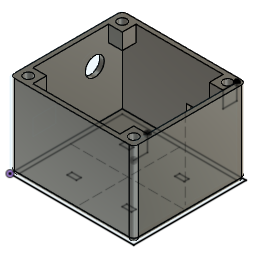
LedstripBox (Autodesk Fusion 360 design; units mm, degrees)
Autodesk Fusion 360 part; units mm, degrees
sketch "Esquisse1" plane through (0, 0, 0) normal (0, 0, 1) x (1, 0, 0)
  line L0 (0, 0) -> (54, 0)
  line L1 (54, 0) -> (54, 49)
  line L2 (54, 49) -> (0, 49)
  line L3 (0, 49) -> (0, 0)
  line L4 (2, 47) -> (52, 47)
  line L5 (52, 47) -> (52, 2)
  line L6 (52, 2) -> (2, 2)
  line L7 (2, 2) -> (2, 47)
  line L8 (13, 37) -> (17, 37)
  line L9 (17, 37) -> (17, 35)
  line L10 (17, 35) -> (13, 35)
  line L11 (13, 35) -> (13, 37)
  line L12 (27, 47) -> (27, 2) construction
  line L13 (2, 24.5) -> (52, 24.5) construction
  line L14 (41, 37) -> (37, 37)
  line L15 (37, 37) -> (37, 35)
  line L16 (37, 35) -> (41, 35)
  line L17 (41, 35) -> (41, 37)
  line L18 (13, 12) -> (17, 12)
  line L19 (13, 14) -> (13, 12)
  line L20 (17, 14) -> (13, 14)
  line L21 (17, 12) -> (17, 14)
  line L22 (37, 12) -> (37, 14)
  line L23 (41, 12) -> (37, 12)
  line L24 (41, 14) -> (41, 12)
  line L25 (37, 14) -> (41, 14)
  dimension "d4" = 54
  dimension "d5" = 49
  dimension "d6" = 2
  dimension "d7" = 2
  dimension "d8" = 2
  dimension "d9" = 2
  dimension "d10" = 4
  dimension "d11" = 2
  dimension "d12" = 10
  dimension "d13" = 10
  constraint horizontal L0
  constraint vertical L1
  constraint horizontal L2
  constraint vertical L3
  constraint coincident L0.start L3.end
  constraint horizontal L4
  constraint vertical L5
  constraint horizontal L6
  constraint vertical L7
  constraint horizontal L8
  constraint vertical L9
  constraint horizontal L10
  constraint vertical L11
  constraint midpoint L4 L12.start
  constraint midpoint L6 L12.end
  constraint midpoint L7 L13.start
  constraint midpoint L5 L13.end
  constraint symmetric L8.start L12 L14.start
  constraint symmetric L8.end L12 L14.end
  constraint symmetric L9.end L12 L15.end
  constraint symmetric L10.end L12 L16.end
  constraint symmetric L8.start L13 L18.start
  constraint symmetric L8.end L13 L18.end
  constraint symmetric L9.end L13 L20.start
  constraint symmetric L10.end L13 L19.start
  constraint symmetric L13 L14.end L22.start
  constraint symmetric L13 L14.start L23.start
  constraint symmetric L13 L15.end L22.end
  constraint symmetric L13 L16.end L24.start
  measures "d4" distance of L0.start L0.end
  measures "d5" distance of L0 L2
  measures "d6" distance of L2 L4
  measures "d7" distance of L3 L7
  measures "d8" distance of L1 L5
  measures "d9" distance of L0 L6
  measures "d10" distance of L8.start L8.end
  measures "d11" distance of L8.start L10.end
  measures "d12" distance of L9 L12
  measures "d13" distance of L4 L8
extrude "Extrusion1" add sketch "Esquisse1" along normal blind 37 contours L0 L1 L2 L3
extrude "Extrusion2" add sketch "Esquisse1" along normal blind 2 contours L4 L5 L6 L7
sketch "Esquisse2" plane through (0, 0, 0) normal (-1, 0, 0) x (0, -1, 0)
  line L0 (-49, 0) -> (0, 0)
  line L1 (0, 0) -> (0, 37)
  line L2 (0, 37) -> (-49, 37)
  line L3 (-49, 37) -> (-49, 0)
  line L4 (-10, 9) -> (-20, 9)
  line L5 (-20, 9) -> (-20, 16)
  line L6 (-20, 16) -> (-10, 16)
  line L7 (-10, 16) -> (-10, 9)
  line L8 (-49, 0) -> (0, 0)
  circle A0 centre (-35, 24) radius 4.125
  dimension "d19" = 10
  dimension "d20" = 7
  dimension "d21" = 9
  dimension "d22" = 10
  dimension "d23" = 8.25
  constraint horizontal L4
  constraint vertical L5
  constraint horizontal L6
  constraint vertical L7
  measures "d19" distance of L4.start L4.end
  measures "d20" distance of L4.start L6.end
  measures "d21" distance of L4 L8
  measures "d22" distance of L1 L7
  measures "d23" diameter of A0
extrude "Extrusion3" cut sketch "Esquisse2" against normal blind 11 contours L4 L5 L6 L7 | A0
sketch "Esquisse3" plane through (0, 49, 0) normal (0, 1, 0) x (-1, 0, 0)
  line L0 (-54, 0) -> (0, 0)
  line L1 (0, 0) -> (0, 37)
  line L2 (0, 37) -> (-54, 37)
  line L3 (-54, 37) -> (-54, 0)
  line L4 (-46, 8) -> (-30, 8)
  line L5 (-30, 8) -> (-30, 18)
  line L6 (-30, 18) -> (-46, 18)
  line L7 (-46, 18) -> (-46, 8)
  point P0 (-41, 0)
  dimension "d26" = 16
  dimension "d27" = 10
  dimension "d28" = 8
  dimension "d29" = 8
  constraint horizontal L4
  constraint vertical L5
  constraint horizontal L6
  constraint vertical L7
  measures "d26" distance of L4.start L4.end
  measures "d27" distance of L4.start L6.end
  measures "d28" distance of L4 P0
  measures "d29" distance of L3 L7
extrude "Extrusion4" cut sketch "Esquisse3" against normal blind 6 contours L4 L5 L6 L7
sketch "Esquisse4" plane through (0, 0, 0) normal (-1, 0, 0) x (0, -1, 0)
  circle A0 centre (-35, 24) radius 4.125
  line L0 (-20, 9) -> (-20, 16)
  line L1 (-20, 16) -> (-10, 16)
  line L2 (-10, 16) -> (-10, 9)
  line L3 (-10, 9) -> (-20, 9)
  line L4 (-49, 0) -> (0, 0)
  line L5 (0, 0) -> (0, 37)
  line L6 (0, 37) -> (-49, 37)
  line L7 (-49, 37) -> (-49, 0)
sketch "Esquisse5" plane through (52, 0, 0) normal (-1, 0, 0) x (0, -1, 0)
  line L0 (-47, 2) -> (-2, 2)
  line L1 (-2, 2) -> (-2, 37)
  line L2 (-2, 37) -> (-47, 37)
  line L3 (-47, 37) -> (-47, 2)
  line L4 (-47, 37) -> (-41, 37)
  line L5 (-41, 37) -> (-41, 30)
  line L6 (-41, 30) -> (-47, 30)
  line L7 (-47, 30) -> (-47, 37)
  line L8 (-24.5, 37) -> (-24.5, 2) construction
  line L9 (-8, 37) -> (-8, 30)
  line L10 (-8, 30) -> (-2, 30)
  dimension "d34" = 7
  dimension "d35" = 6
  constraint horizontal L4
  constraint vertical L5
  constraint horizontal L6
  constraint vertical L7
  constraint coincident L2.end L3.start
  constraint midpoint L2 L8.start
  constraint midpoint L0 L8.end
  constraint symmetric L4.end L8 L9.start
  constraint symmetric L5.end L8 L9.end
  constraint symmetric L6.end L8 L10.end
  measures "d34" distance of L4 L6
  measures "d35" distance of L5 L7
extrude "Extrusion5" add sketch "Esquisse5" along normal blind 6 contours L2 L3 L4 L5 L6 L7 | L1 L2 L9 L10
sketch "Esquisse6" plane through (2, 0, 0) normal (1, 0, 0) x (0, 1, 0)
  circle A0 centre (35, 24) radius 4.125
  line L0 (20, 16) -> (20, 9)
  line L1 (20, 9) -> (10, 9)
  line L2 (10, 9) -> (10, 16)
  line L3 (10, 16) -> (20, 16)
  line L4 (2, 2) -> (47, 2)
  line L5 (47, 2) -> (47, 37)
  line L6 (47, 37) -> (2, 37)
  line L7 (2, 37) -> (2, 2)
  line L8 (2, 37) -> (8, 37)
  line L9 (8, 37) -> (8, 30)
  line L10 (8, 30) -> (2, 30)
  line L11 (2, 30) -> (2, 37)
  line L12 (24.5, 37) -> (24.5, 2) construction
  line L13 (41, 37) -> (41, 30)
  line L14 (41, 30) -> (47, 30)
  dimension "d36" = 6
  dimension "d37" = 7
  constraint horizontal L8
  constraint vertical L9
  constraint horizontal L10
  constraint vertical L11
  constraint coincident L6.end L7.start
  constraint midpoint L6 L12.start
  constraint midpoint L4 L12.end
  constraint symmetric L8.end L12 L13.start
  constraint symmetric L9.end L12 L13.end
  constraint symmetric L10.end L12 L14.end
  measures "d36" distance of L6.end L8.end
  measures "d37" distance of L6.end L10.end
extrude "Extrusion6" add sketch "Esquisse6" along normal blind 6 contours L6 L7 L8 L9 L10 L11 | L5 L6 L13 L14
fillet "Congé1" radius 2 8 edges at (54, 49, 18.5) (0, 0, 18.5) (0, 49, 18.5) (54, 0, 18.5) (54, 24.5, 0) (27, 0, 0) (27, 49, 0) (0, 24.5, 0)
sketch "Esquisse7" plane through (0, 0, 37) normal (0, 0, 1) x (-1, 0, 0)
  line L0 (-46, -2) -> (-8, -2)
  line L1 (-8, -2) -> (-8, -8)
  line L2 (-8, -8) -> (-2, -8)
  line L3 (-2, -8) -> (-2, -41)
  line L4 (-2, -41) -> (-8, -41)
  line L5 (-8, -41) -> (-8, -47)
  line L6 (-8, -47) -> (-46, -47)
  line L7 (-46, -47) -> (-46, -41)
  line L8 (-46, -41) -> (-52, -41)
  line L9 (-52, -41) -> (-52, -8)
  line L10 (-52, -8) -> (-46, -8)
  line L11 (-46, -8) -> (-46, -2)
  arc A0 (0, -2) -> (-2, 0) centre (-2, -2) ccw
  line L12 (-2, 0) -> (-52, 0)
  arc A1 (-52, 0) -> (-54, -2) centre (-52, -2) ccw
  line L13 (-54, -2) -> (-54, -47)
  arc A2 (-54, -47) -> (-52, -49) centre (-52, -47) ccw
  line L14 (-52, -49) -> (-2, -49)
  arc A3 (-2, -49) -> (0, -47) centre (-2, -47) ccw
  line L15 (0, -47) -> (0, -2)
  line L16 (-4, -41) -> (-4, -49) construction
  line L17 (0, -49) -> (0, 0) construction
  line L18 (0, -45) -> (-8, -45) construction
  line L19 (-54, -49) -> (0, -49) construction
  circle A4 centre (-4, -45) radius 2
  line L20 (-27, -49) -> (-27, 0) construction
  line L21 (0, -24.5) -> (-54, -24.5) construction
  circle A5 centre (-50, -45) radius 2
  circle A6 centre (-4, -4) radius 2
  circle A7 centre (-50, -4) radius 2
  dimension "d45" = 4
  constraint coincident L4 L16.start
  constraint coincident L14 L16.end
  constraint perpendicular L14 L16
  constraint coincident L15 L18.start
  constraint coincident L5 L18.end
  constraint perpendicular L5 L18
  constraint midpoint L18 A4.centre
  constraint midpoint L19 L20.start
  constraint midpoint L12 L20.end
  constraint midpoint L17 L21.start
  constraint midpoint L13 L21.end
  constraint symmetric A4 L20 A5
  constraint symmetric A4 L21 A6
  constraint symmetric L21 A5 A7
  measures "d45" diameter of A4
extrude "Extrusion7" cut sketch "Esquisse7" against normal blind 6 contours A4 | A5 | A6 | A7
equation "BoardWidth = 52 mm"
equation "BoardLength = 47 mm"
equation "walls = 2 mm"
equation "d4 = BoardWidth + walls"
equation "d5 = BoardLength + walls"
equation "d6 = walls"
equation "d7 = walls"
equation "d8 = walls"
equation "d9 = walls"
equation "Hauteur = 35 mm"
equation "d15 = Hauteur + walls"
equation "d17 = walls"
equation "d21 = 7.00 mm + walls"
equation "d22 = 8 mm + walls"
